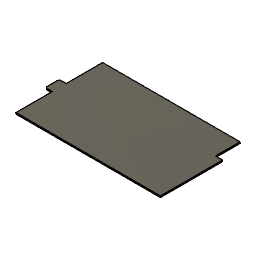
Control board - middle plate v2 (Autodesk Fusion 360 design; units mm, degrees)
Autodesk Fusion 360 part; units mm, degrees
sketch "Sketch1" plane through (0, 0, 0) normal (0, 0, 1) x (1, 0, 0)
  line L0 (3.6667, 54.4476) -> (106.5667, 54.4476)
  line L1 (106.5667, 54.4476) -> (106.5667, -7.3524)
  line L2 (106.5667, -7.3524) -> (3.6667, -7.3524)
  line L3 (3.6667, -7.3524) -> (3.6667, 54.4476)
  line L4 (3.6667, 23.5476) -> (106.5667, 23.5476) construction
  line L5 (3.6667, 28.5476) -> (-0.0333, 28.5476)
  line L6 (-1.3333, 27.2476) -> (-1.3333, 19.8476)
  line L7 (-0.0333, 18.5476) -> (3.6667, 18.5476)
  line L8 (3.6667, 18.5476) -> (3.6667, 28.5476)
  arc A0 (-0.0333, 28.5476) -> (-1.3333, 27.2476) centre (-0.0333, 27.2476) ccw
  arc A1 (-1.3333, 19.8476) -> (-0.0333, 18.5476) centre (-0.0333, 19.8476) ccw
  line L9 (101.5667, 54.4476) -> (106.5667, 54.4476)
  line L10 (106.5667, 54.4476) -> (106.5667, 36.9476)
  line L11 (106.5667, 36.9476) -> (101.5667, 36.9476)
  line L12 (101.5667, 36.9476) -> (101.5667, 54.4476)
  point P0 (-1.3333, 28.5476)
  point P1 (-1.3333, 18.5476)
  dimension "d1" = 102.9
  dimension "d2" = 61.8
  dimension "d7" = 10
  dimension "d8" = 5
  dimension "d9" = 1.3
  dimension "d12" = 5
  dimension "d13" = 17.5
  constraint horizontal L0
  constraint vertical L1
  constraint horizontal L2
  constraint vertical L3
  constraint midpoint L3 L4.start
  constraint midpoint L1 L4.end
  constraint horizontal L5
  constraint vertical L6
  constraint horizontal L7
  constraint vertical L8
  constraint coincident L3 L5.start
  constraint symmetric L4 L5 L7
  constraint coincident P0 L5
  constraint coincident P0 L6
  constraint tangent L5 A0
  constraint tangent L6 A0
  constraint coincident P1 L6
  constraint coincident P1 L7
  constraint tangent L6 A1
  constraint tangent L7 A1
  constraint equal A0 A1
  constraint horizontal L9
  constraint vertical L10
  constraint horizontal L11
  constraint vertical L12
  constraint coincident L1 L10.end
  constraint coincident L0 L9.start
  measures "d1" distance of L0.start L0.end
  measures "d2" distance of L0.end L1.end
  measures "d7" distance of P0 P1
  measures "d8" distance of L5.start P0
  measures "d9" radius of A0
  measures "d12" distance of L10 L12
  measures "d13" distance of L9 L11
extrude "Extrude1" add sketch "Sketch1" along normal blind 1 contours L0 L1 L2 L3 L8 L11 L12 | L3 L5 L6 L7 L8 A0 A1
